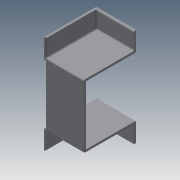
# Autodesk Inventor part: servodrzak0
Saved by Autodesk Inventor 2013 (Build 170138000, 138)
## iProperties
Created: 2013-01-30
Part Number: servodrzak0
Material: Generic
Document SubType Name: Modeling
Designer: idle-rug
Density: 1 g/cm^3
Author: idle-rug
Autodesk Inventor part; units mm, degrees
ref_plane "YZ Plane" through (0, 0, 0) normal (1, 0, 0) x (0, 1, 0)
ref_plane "XZ Plane" through (0, 0, 0) normal (0, 1, 0) x (-1, 0, 0)
ref_plane "XY Plane" through (0, 0, 0) normal (0, 0, 1) x (1, 0, 0)
sketch "Sketch1" plane through (0, 0, 0) normal (0, 1, 0) x (-1, 0, 0)
  line L0 (13.9, 22.1) -> (-13.9, 22.1)
  line L1 (-13.9, 22.1) -> (-13.9, -22.1)
  line L2 (-13.9, -22.1) -> (13.9, -22.1)
  line L3 (13.9, -22.1) -> (13.9, 22.1)
  line L4 (13.9, 22.1) -> (-13.9, -22.1) construction
  line L5 (-13.9, 22.1) -> (13.9, -22.1) construction
  point P0 (0, 0)
  dimension "d0" = 27.8
  dimension "d1" = 44.2
  constraints: 12 end point, 2 midpoint, 2 parallel, 1 horizontal, 1 perpendicular
  measures "d0" distance of L2.end L1.end
  measures "d1" distance of L1.end L0.end
extrude "Extrusion1" add sketch "Sketch1" along normal blind 1.5
sketch "Sketch2" plane through (0, 1.5, 0) normal (0, 1, 0) x (1, 0, 0)
  line L0 (-13.9, -22.1) -> (13.9, -22.1) projected
  line L1 (13.9, 22.1) -> (-13.9, 22.1) projected
  line L2 (-13.9, 22.1) -> (-13.9, 20.6)
  line L3 (-13.9, 20.6) -> (13.9, 20.6)
  line L4 (-13.9, -22.1) -> (-13.9, -20.6)
  line L5 (-13.9, -20.6) -> (13.9, -20.6)
  line L6 (13.9, 20.6) -> (13.9, 22.1)
  line L7 (13.9, -20.6) -> (13.9, -22.1)
  point P0 (0, 0)
  dimension "d4" = 1.5
  dimension "d5" = 1.5
  constraints: 12 end point
  measures "d4" distance of L1.end L2.end
  measures "d5" distance of L0.start L4.end
extrude "Extrusion2" add sketch "Sketch2" along normal blind 35
sketch "Sketch3" plane through (-13.9, 0, 22.1) normal (0, 0, 1) x (1, 0, 0)
  line L0 (0, 36.5) -> (27.8, 36.5) projected
  line L1 (0, 36.5) -> (0, 35)
  line L2 (0, 35) -> (27.8, 35)
  line L3 (27.8, 36.5) -> (27.8, 35)
  point P0 (13.9, 0)
  dimension "d8" = 1.5
  constraints: 6 end point
  measures "d8" distance of L0.start L1.end
sketch "Sketch4" plane through (13.9, 0, -22.1) normal (0, 0, -1) x (-1, 0, 0)
  line L0 (0, 36.5) -> (27.8, 36.5) projected
  line L1 (0, 36.5) -> (0, 35)
  line L2 (0, 35) -> (27.8, 35)
  line L3 (27.8, 36.5) -> (27.8, 35)
  dimension "d9" = 1.5
  constraints: 6 end point, 1 perpendicular
  measures "d9" distance of L0.start L1.end
extrude "Extrusion3" add sketch "Sketch4" along normal blind 12
extrude "Extrusion4" add sketch "Sketch3" along normal blind 12
sketch "Sketch5" plane through (-13.9, 0, -22.1) normal (-1, 0, 0) x (0, 0, 1)
  line L0 (44.2, 0) -> (44.2, 35) projected
  line L1 (44.2, 35) -> (56.2, 35) projected
  line L2 (56.2, 36.5) -> (56.2, 35) projected
  line L3 (42.7, 36.5) -> (56.2, 36.5) projected
  line L4 (42.7, 1.5) -> (42.7, 36.5) projected
  line L5 (1.5, 1.5) -> (1.5, 36.5) projected
  line L6 (1.5, 36.5) -> (-12, 36.5) projected
  line L7 (-12, 35) -> (-12, 36.5) projected
  line L8 (0, 35) -> (-12, 35) projected
  line L9 (0, 0) -> (0, 35) projected
  line L10 (1.5, 1.5) -> (1.5, 0)
  line L11 (1.5, 0) -> (0, 0)
  line L12 (42.7, 1.5) -> (42.7, 0)
  line L13 (42.7, 0) -> (44.2, 0)
  constraints: 8 end point, 3 perpendicular, 1 parallel
extrude "Extrusion5" add sketch "Sketch5" along normal blind 1.5
sketch "Sketch6" plane through (13.9, 0, 22.1) normal (0, 0, 1) x (1, 0, 0)
  line L0 (0, 35) -> (-29.3, 35) projected
  line L1 (-29.3, 0) -> (-29.3, 35) projected
  line L2 (-29.3, 0) -> (0, 0) projected
  line L3 (-29.3, 35) -> (-27.8, 35)
  line L4 (-27.8, 35) -> (-27.8, 0)
  line L5 (-29.3, 0) -> (-27.8, 0)
  point P0 (-13.9, 0)
  dimension "d16" = 1.5
  constraints: 6 end point, 2 point on line, 1 collinear, 1 perpendicular
  measures "d16" distance of L0.end L3.end
extrude "Extrusion6" add sketch "Sketch6" along normal blind 12
sketch "Sketch7" plane through (13.9, 0, -22.1) normal (0, 0, -1) x (-1, 0, 0)
  line L0 (29.3, 35) -> (0, 35) projected
  line L1 (0, 0) -> (29.3, 0) projected
  line L2 (29.3, 35) -> (29.3, 0) projected
  line L3 (29.3, 35) -> (27.8, 35)
  line L4 (27.8, 35) -> (27.8, 0)
  line L5 (29.3, 0) -> (27.8, 0)
  point P0 (13.9, 0)
  dimension "d19" = 1.5
  constraints: 6 end point, 2 point on line, 1 collinear, 1 perpendicular
  measures "d19" distance of L0.start L3.end
extrude "Extrusion7" add sketch "Sketch7" along normal blind 12
fillet "Fillet1" radius 1 4 edges at (-15.4, 18.25, 20.6) (-15.4, 18.25, -20.6) (-13.9, 17.5, 22.1) (-13.9, 17.5, -34.1)
fillet "Fillet2" radius 1 15 edges at (0, 0, -22.1) (-13.6071, 0, 22.3929) (-13.9, 0, 28.6) (0.5, 0, 22.1) (0, 35, 34.1) (-13.6071, 35, 22.3929) (-13.9, 35, 28.6) (0.5, 35, 22.1) (0, 35, -22.1) (-15.1071, 36.5, -20.8929) (-0.25, 36.5, -20.6) (-15.4, 36.5, -27.85) (-0.25, 36.5, 20.6) (-15.4, 36.5, 27.85) (-15.1071, 36.5, 20.8929)
sketch "Sketch8" plane through (13.9, 1.5, 20.6) normal (1, 0, 0) x (0, 0, -1)
  arc A0 (0, 34) -> (-1, 35) centre (-1, 34) ccw projected
  line L0 (-1, 35) -> (-13.5, 35) projected
  line L1 (-13.5, 34.5) -> (-13.5, 35) projected
  arc A1 (-13.5, 34.5) -> (-12.5, 33.5) centre (-12.5, 34.5) ccw projected
  line L2 (-2.5, 33.5) -> (-12.5, 33.5) projected
  arc A2 (-1.5, 32.5) -> (-2.5, 33.5) centre (-2.5, 32.5) ccw projected
  line L3 (-1.5, -0.5) -> (-1.5, 32.5) projected
  arc A3 (-1.5, -0.5) -> (-0.5, -1.5) centre (-0.5, -0.5) ccw projected
  line L4 (-0.5, -1.5) -> (41.7, -1.5) projected
  arc A4 (41.7, -1.5) -> (42.7, -0.5) centre (41.7, -0.5) ccw projected
  line L5 (42.7, -0.5) -> (42.7, 32.5) projected
  arc A5 (43.7, 33.5) -> (42.7, 32.5) centre (43.7, 32.5) ccw projected
  line L6 (43.7, 33.5) -> (54.7, 33.5) projected
  line L7 (54.7, 35) -> (54.7, 33.5) projected
  line L8 (42.2, 35) -> (54.7, 35) projected
  arc A6 (42.2, 35) -> (41.2, 34) centre (42.2, 34) ccw projected
  line L9 (41.2, 0) -> (41.2, 34) projected
  line L10 (0, 0) -> (41.2, 0) projected
  line L11 (0, 0) -> (0, 34) projected
  point P0 (20.6, -1.5)
extrude "Extrusion8" cut sketch "Sketch8" against normal blind 1.5
body "Solid1"
